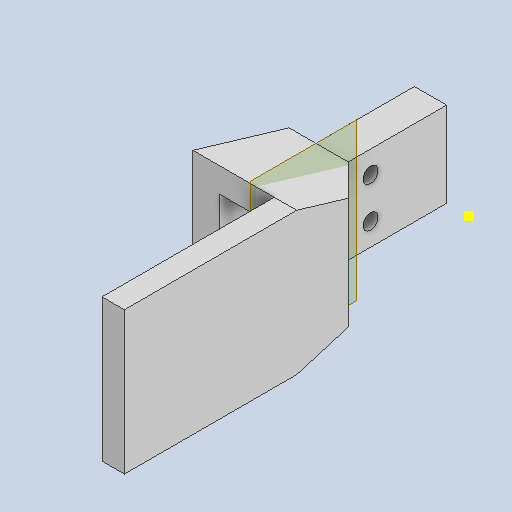
# Autodesk Inventor part: Finger
Saved by Autodesk Inventor 2022 (Build 260153000, 153)
## iProperties
Created: 2021-09-24
Part Number: Finger
Material: Generic
Document SubType Name: Modeling
Designer: kylem
Density: 1 g/cm^3
Appearance: Default
Author: kylem
Autodesk Inventor part; units mm, degrees
ref_plane "YZ Plane" through (0, 0, 0) normal (1, 0, 0) x (0, 1, 0)
ref_plane "XZ Plane" through (0, 0, 0) normal (0, 1, 0) x (-1, 0, 0)
ref_plane "XY Plane" through (0, 0, 0) normal (0, 0, 1) x (1, 0, 0)
sketch "Sketch1" plane through (0, 0, 0) normal (1, 0, 0) x (0, 1, 0)
  line L0 (0, 0) -> (19, 0)
  line L1 (19, 0) -> (19, 22)
  line L2 (19, 22) -> (0, 22)
  line L3 (0, 22) -> (0, 0)
  line L4 (19, 22) -> (14, 22)
  line L5 (14, 22) -> (14, 17)
  line L6 (14, 17) -> (19, 17)
  line L7 (19, 17) -> (19, 22)
  line L8 (0, 22) -> (5, 22)
  line L9 (5, 22) -> (5, 17)
  line L10 (5, 17) -> (0, 17)
  line L11 (0, 17) -> (0, 22)
  circle A0 centre (14, 17) radius 1.7
  circle A1 centre (5, 17) radius 1.7
  dimension "d0" = 19
  dimension "d1" = 22
  dimension "d2" = 5
  dimension "d3" = 5
  dimension "d4" = 5
  dimension "d5" = 5
  dimension "d6" = 3.4
  dimension "d7" = 3.4
  constraints: 24 end point, 6 parallel, 3 horizontal, 3 perpendicular, 2 centre point, 2 coincident
  measures "d0" distance of L2.end L1.end
  measures "d1" distance of L1.end L0.end
  measures "d2" distance of L6.end L5.end
  measures "d3" distance of L5.end L4.end
  measures "d4" distance of L9.end L10.end
  measures "d5" distance of L8.end L9.end
  measures "d6" diameter of A0
  measures "d7" diameter of A1
extrude "Extrusion1" add sketch "Sketch1" along normal blind 17.2 contours L3 L10 A1 L9 L2 L5 A0 L6 L1 L0 | L3 L2 L9 A1 L10 | L6 A0 L5 L2 L1
sketch "Sketch2" plane through (0, 19, 22) normal (0, 1, 0) x (1, 0, 0)
  line L0 (0, 0) -> (17.2, 0) projected
  line L1 (17.2, 0) -> (-6, 0)
  line L2 (-6, 0) -> (-6, -60)
  line L3 (-6, -60) -> (17.2, -60)
  line L4 (17.2, -60) -> (17.2, 0)
  point P0 (0, 22)
  dimension "d10" = 23.2
  dimension "d11" = 60
  constraints: 8 end point, 2 parallel, 1 horizontal, 1 perpendicular
  measures "d10" distance of L3.end L2.end
  measures "d11" distance of L2.end L1.end
extrude "Extrusion2" add sketch "Sketch2" against normal blind 19
sketch "Sketch3" plane through (-6, 19, 22) normal (-1, 0, 0) x (0, 0, 1)
  line L0 (-22, 0) -> (60, 0) projected
  line L1 (-22, -19) -> (60, -19) projected
  line L2 (60, 0) -> (21.5, 0)
  line L3 (21.5, 0) -> (21.5, -19)
  line L4 (21.5, -19) -> (60, -19)
  line L5 (60, -19) -> (60, 0)
  point P0 (-10, 0)
  point P1 (-10, -19)
  dimension "d23" = 38.5
  constraints: 8 end point, 2 parallel, 1 horizontal, 1 perpendicular, 1 point on line
  measures "d23" distance of L4.end L3.end
extrude "Extrusion3" cut sketch "Sketch3" against normal blind 18.2
sketch "Sketch4" plane through (17.2, 0, 0) normal (1, 0, 0) x (0, 0, -1)
  line L0 (0, 0) -> (0, 19) projected
  line L1 (0, 19) -> (-82, 19) projected
  line L2 (0, 0) -> (-22, 0)
  line L3 (-22, 0) -> (-22, 19)
  line L4 (-22, 19) -> (0, 19)
  line L5 (0, 19) -> (0, 0)
  dimension "d26" = 22
  constraints: 8 end point, 2 parallel, 1 horizontal, 1 perpendicular, 1 point on line
  measures "d26" distance of L3.end L4.end
extrude "Extrusion4" cut sketch "Sketch4" against normal blind 10
sketch "Sketch5" plane through (17.2, 0, 0) normal (1, 0, 0) x (0, 0, -1)
  line L0 (-22, 0) -> (-22, 19) projected
  line L1 (-22, 9.5) -> (-22, 25.4)
  line L2 (-43.5, 0) -> (-43.5, 19) projected
  line L3 (-22, 25.4) -> (-43.5, 25.4)
  line L4 (-43.5, 25.4) -> (-43.5, 19)
  line L5 (-43.5, 19) -> (-22, 19)
  line L6 (-22, 19) -> (-22, 25.4)
  line L7 (0, 19) -> (-22, 19) projected
  line L8 (-43.5, 25.4) -> (-22, 19)
  line L9 (-22, 9.5) -> (-27.2776, 9.5)
  line L10 (-22, 19) -> (-22, 0)
  line L11 (-22, 9.5) -> (-22, -6.4)
  line L12 (-43.5, 19) -> (-43.5, 0)
  line L13 (-22, -6.4) -> (-43.5, -6.4)
  line L14 (-43.5, -6.4) -> (-43.5, 0)
  line L15 (-43.5, 0) -> (-22, 0)
  line L16 (-22, 0) -> (-22, -6.4)
  line L17 (0, 0) -> (-22, 0)
  line L18 (-43.5, -6.4) -> (-22, 0)
  point P0 (0, 0)
  dimension "d29" = 15.9
  constraints: 32 end point, 8 symmetric about line, 2 horizontal, 2 parallel, 1 collinear, 1 midpoint, 1 perpendicular
  measures "d29" distance of L1.start L1.end
extrude "Extrusion5" add sketch "Sketch5" against normal blind 23.2 contours L18 L14 L15 | L5 L4 L8
sketch "Sketch6" plane through (17.2, 0, 0) normal (1, 0, 0) x (0, 0, -1)
  line L0 (-82, 19) -> (-82, 0) projected
  line L1 (-43.5, -6.4) -> (-43.5, 25.4) projected
  line L2 (-82, 0) -> (-43.5, 0)
  line L3 (-43.5, 0) -> (-43.5, -6.4)
  line L4 (-43.5, -6.4) -> (-82, -6.4)
  line L5 (-82, -6.4) -> (-82, 0)
  line L6 (-43.5, 19) -> (-82, 19) projected
  line L7 (-43.5, 25.4) -> (-22, 19) projected
  line L8 (-82, 19) -> (-43.5, 19)
  line L9 (-43.5, 19) -> (-43.5, 25.4)
  line L10 (-43.5, 25.4) -> (-82, 25.4)
  line L11 (-82, 25.4) -> (-82, 19)
  point P0 (0, 0)
  constraints: 16 end point, 4 parallel, 2 horizontal, 2 perpendicular
extrude "Extrusion6" add sketch "Sketch6" against normal blind 5 contours L11 L10 L1 L6 | L2 L1 L4 L5
chamfer "Chamfer4" distance 10 angle 45 1 edges at (17.2, 9.5, 22)
ref_plane "Work Plane1" through (8, -6.4, 43.5) normal (-1, 0, 0) x (0, 0, 1)
sketch "Sketch11" plane through (8, -6.4, 43.5) normal (-1, 0, 0) x (0, 0, 1)
  line L0 (38.5, 31.8) -> (0, 31.8) projected
  line L1 (38.5, 0) -> (0, 0) projected
  line L2 (0, 31.8) -> (0, 0)
  line L3 (0, 0) -> (0, 31.8) projected
  line L4 (0, 15.9) -> (0, 5.5)
  line L5 (0, 5.5) -> (0, 26.3)
  line L6 (0, 26.3) -> (-14, 26.3)
  line L7 (-14, 26.3) -> (-19.2094, -3.2442)
  line L8 (0, 5.5) -> (-2, 5.5)
  line L9 (-2, 5.5) -> (-2, -4.5)
  line L10 (-19.2094, -3.2442) -> (-2, -4.5)
  point P0 (-43.5, 6.4)
  dimension "d61" = 10.4
  dimension "d62" = 20.8
  dimension "d63" = 14
  dimension "d64" = 30
  dimension "d65" = 100
  dimension "d66" = 2
  dimension "d67" = 10
  dimension "d68" = 90
  constraints: 16 end point, 2 perpendicular, 2 point on line, 1 midpoint, 1 vertical
  measures "d61" distance of L4.start L4.end
  measures "d62" distance of L4.end L5.end
  measures "d63" distance of L5.end L6.end
  measures "d64" distance of L6.end L7.end
  measures "d65" angle of L7 L6
  measures "d66" distance of L4.end L8.end
  measures "d67" distance of L8.end L9.end
  measures "d68" angle of L9 L8
extrude "Extrusion10" cut sketch "Sketch11" along normal blind 8
sketch "Sketch12" plane through (12.2, 19, 22) normal (-1, 0, 0) x (0, 0, 1)
  point P0 (-22, -19)
body "Solid1"
